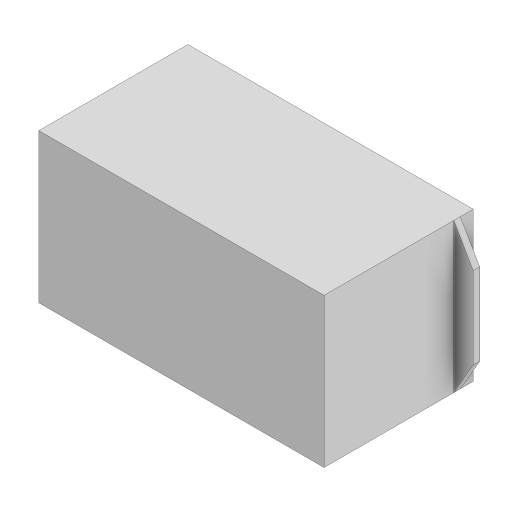
# Autodesk Inventor part: кейсик
Saved by Autodesk Inventor 2023.2 (Build 272271000, 271)
## iProperties
Created: 2023-11-25
Part Number: кейсик
Material: Типовые
Document SubType Name: Modeling
Designer: matvey
Density: 1 g/cm^3
Appearance: По умолчанию
Author: matvey
Autodesk Inventor part; units mm, degrees
ref_plane "YZ Plane" through (0, 0, 0) normal (1, 0, 0) x (0, 1, 0)
ref_plane "XZ Plane" through (0, 0, 0) normal (0, 1, 0) x (-1, 0, 0)
ref_plane "XY Plane" through (0, 0, 0) normal (0, 0, 1) x (1, 0, 0)
sketch "Эскиз1" plane through (0, 0, 0) normal (0, 0, 1) x (1, 0, 0)
  line L0 (22, -11.5) -> (-22, -11.5)
  line L1 (-22, -11.5) -> (-22, 11.5)
  line L2 (-22, 11.5) -> (22, 11.5)
  line L3 (22, 11.5) -> (22, -11.5)
  line L4 (22, -11.5) -> (-22, 11.5) construction
  line L5 (-22, -11.5) -> (22, 11.5) construction
  line L6 (20, -10.4545) -> (-20, 10.4545) construction
  line L7 (-20, -10.4545) -> (20, 10.4545) construction
  line L8 (21, -10.5) -> (-21, -10.5)
  line L9 (-21, -10.5) -> (-21, 10.5)
  line L10 (-21, 10.5) -> (21, 10.5)
  line L11 (21, 10.5) -> (21, -10.5)
  line L12 (21, -10.5) -> (-21, 10.5) construction
  line L13 (-21, -10.5) -> (21, 10.5) construction
  point P0 (0, 0)
  dimension "d0" = 23
  dimension "d1" = 44
  dimension "d3" = 1
  dimension "d4" = 1
  dimension "d5" = 1
  constraints: 28 end point, 6 midpoint, 4 parallel, 2 horizontal, 2 perpendicular, 1 point on line
  measures "d0" distance between parallel lines of L0 L2
  measures "d1" distance between parallel lines of L3 L1
  measures "d3" distance between parallel lines of L10 L2
  measures "d4" distance between parallel lines of L0 L8
  measures "d5" distance between parallel lines of L3 L11
extrude "Выдавливание1" add sketch "Эскиз1" along normal blind 20
sketch "Эскиз3" plane through (0, 0, 20) normal (0, 0, 1) x (1, 0, 0)
  line L0 (22, 11.5) -> (-22, 11.5) projected
  line L1 (-22, -11.5) -> (22, -11.5) projected
  line L2 (-22, 11.5) -> (22, 11.5)
  line L3 (22, 11.5) -> (22, -11.5)
  line L4 (22, -11.5) -> (-22, -11.5)
  line L5 (-22, -11.5) -> (-22, 11.5)
  point P0 (0, 0)
  constraints: 8 end point, 2 parallel, 1 horizontal, 1 perpendicular
extrude "Выдавливание2" add sketch "Эскиз3" along normal blind 1
sketch "Эскиз4" plane through (0, 0, 0) normal (0, 0, -1) x (-1, 0, 0)
  line L0 (25, -6.3038) -> (25, 6.3038)
  line L1 (-22, 11.5) -> (22, 11.5) projected
  line L2 (25, 6.3038) -> (22, 11.5)
  line L3 (22, -11.5) -> (-22, -11.5) projected
  line L4 (22, 11.5) -> (22, -11.5)
  line L5 (22, -11.5) -> (25, -6.3038)
  line L6 (-22, -11.5) -> (-22, 11.5) projected
  line L7 (-22, -11.5) -> (-22, 11.5)
  line L8 (-22, 11.5) -> (-25, 6.3038)
  line L9 (-25, 6.3038) -> (-25, -6.3038)
  line L10 (-25, -6.3038) -> (-22, -11.5)
  point P0 (0, 0)
  dimension "d10" = 3
  dimension "d11" = 3
  dimension "d12" = 30
  dimension "d13" = 30
  dimension "d14" = 30
  dimension "d15" = 30
  constraints: 16 end point, 2 vertical, 1 parallel, 1 perpendicular
  measures "d10" distance between parallel lines of L4 L0
  measures "d11" distance between parallel lines of L6 L9
  measures "d12" angle of L4 L5
  measures "d13" angle of L4 L2
  measures "d14" angle of L6 L10
  measures "d15" angle of L6 L8
extrude "Выдавливание3" add sketch "Эскиз4" against normal blind 1 contours L5 L4 L2 L0 | L10 L9 L8 L6
sketch "Эскиз5" plane through (0, 0, 0) normal (0, 0, -1) x (-1, 0, 0)
  line L0 (-21, 10.5) -> (-21, -10.5) projected
  line L1 (-21, -10.5) -> (21, -10.5) projected
  line L2 (21, -10.5) -> (21, 10.5) projected
  line L3 (21, 10.5) -> (-21, 10.5) projected
  line L4 (22, -11.5) -> (-22, -11.5)
  line L5 (-22, -11.5) -> (-22, 11.5)
  line L6 (-22, 11.5) -> (22, 11.5)
  line L7 (22, 11.5) -> (22, -11.5)
  point P0 (0, 0)
  constraints: 8 end point, 3 other
extrude "Выдавливание4" add sketch "Эскиз5" along normal blind 2
